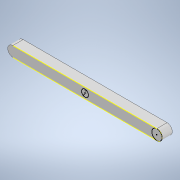
# Autodesk Inventor part: u_kleine_Hoehenverstellung
Saved by Autodesk Inventor 2020.3 (Build 243373000, 373)
## iProperties
Created: 2020-10-04
Part Number: u_kleine_Hoehenverstellung
Material: Generic
Document SubType Name: Modeling
Designer: Mara
Density: 1 g/cm^3
Appearance: Default
Author: Mara
Autodesk Inventor part; units mm, degrees
ref_plane "YZ Plane" through (0, 0, 0) normal (1, 0, 0) x (0, 1, 0)
ref_plane "XZ Plane" through (0, 0, 0) normal (0, 1, 0) x (-1, 0, 0)
ref_plane "XY Plane" through (0, 0, 0) normal (0, 0, 1) x (1, 0, 0)
sketch "Sketch1" plane through (0, 0, 0) normal (0, 0, 1) x (1, 0, 0)
  line L0 (-210, -15) -> (210, -15)
  line L1 (210, -15) -> (210, 15) construction
  line L2 (210, 15) -> (-210, 15)
  line L3 (-210, 15) -> (-210, -15) construction
  line L4 (-210, -15) -> (210, 15) construction
  line L5 (210, -15) -> (-210, 15) construction
  arc A0 (-210, 15) -> (-210, -15) centre (-210, 0) ccw
  arc A1 (210, -15) -> (210, 15) centre (210, 0) ccw
  point P0 (0, 0)
  dimension "d0" = 420
  dimension "d1" = 30
  constraints: 12 end point, 4 midpoint, 4 point on circle, 2 centre point, 2 parallel, 1 horizontal, 1 perpendicular
  measures "d0" distance of L2.end L1.end
  measures "d1" distance of L0.end L1.end
extrude "Extrusion1" add sketch "Sketch1" along normal blind 30
sketch "Sketch2" plane through (0, 0, 30) normal (0, 0, 1) x (1, 0, 0)
  circle A0 centre (0, 0) radius 10
  line L0 (210, 15) -> (-210, 15) projected
  circle A1 centre (210, 0) radius 15
  line L1 (-210, -15) -> (210, -15) projected
  arc A2 (210, -15) -> (210, 15) centre (210, 0) ccw projected
  dimension "d4" = 20
  constraints: 2 coincident, 2 horizontal, 1 centre point, 1 vertical alignment, 1 other
  measures "d4" diameter of A0
body "Solid1"
